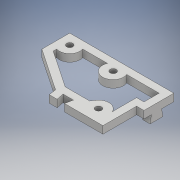
# Autodesk Inventor part: Frame VG01-1
Saved by Autodesk Inventor 2017 (Build 210142000, 142)
## iProperties
Created: 2019-03-04
Part Number: Frame VG01-1
Material: Generic
Document SubType Name: Modeling
Designer: Ben
Density: 1 g/cm^3
Appearance: Default
Author: Ben
Autodesk Inventor part; units mm, degrees
ref_plane "YZ Plane" through (0, 0, 0) normal (1, 0, 0) x (0, 1, 0)
ref_plane "XZ Plane" through (0, 0, 0) normal (0, 1, 0) x (-1, 0, 0)
ref_plane "XY Plane" through (0, 0, 0) normal (0, 0, 1) x (1, 0, 0)
sketch "Sketch1" plane through (0, 0, 0) normal (0, 1, 0) x (-1, 0, 0)
  line L0 (0, 0) -> (0, -35)
  line L1 (0, -35) -> (37, -35)
  line L2 (37, -35) -> (37, -55)
  line L3 (37, -55) -> (48, -55)
  line L4 (48, -55) -> (48, 0)
  line L5 (48, 0) -> (22, 0)
  line L6 (22, 0) -> (22, 0)
  line L7 (22, 0) -> (0, 0)
  dimension "d0" = 35
  dimension "d1" = 37
  dimension "d2" = 20
  dimension "d3" = 11
  dimension "d4" = 55
  dimension "d5" = 26
  dimension "d6" = 0
  constraints: 16 end point, 5 perpendicular, 2 vertical
  measures "d0" distance of L0.start L0.end
  measures "d1" distance of L0.end L1.end
  measures "d2" distance of L1.end L2.end
  measures "d3" distance of L2.end L3.end
  measures "d4" distance of L3.end L4.end
  measures "d5" distance of L4.end L5.end
  measures "d6" distance of L5.end L6.end
extrude "Extrusion1" add sketch "Sketch1" along normal blind 50
shell "Shell1" thickness 5 removed faces 3 at (-19.6667, 0, -23.3333) at (-48, 16.6667, -36.6667) at (-19.6667, 50, -23.3333)
sketch "Sketch2" plane through (0, 0, 0) normal (1, 0, 0) x (0, 0, -1)
  line L0 (5, 0) -> (30, 0) projected
  line L1 (5, 0) -> (19, 0)
  line L2 (19, 0) -> (19, 17)
  line L3 (19, 17) -> (5, 17)
  line L4 (5, 17) -> (5, 0)
  point P0 (0, 0)
  dimension "d10" = 17
  dimension "d11" = 0
  dimension "d12" = 11
  constraints: 8 end point, 2 parallel, 1 horizontal, 1 perpendicular, 1 point on line
  measures "d10" distance of L2.end L1.end
  measures "d11" distance from line of L4 L0.start
  measures "d12" distance from line of L2 L0.end
extrude "Extrusion2" cut sketch "Sketch2" against normal blind 10
sketch "Sketch3" plane through (-48, 0, -55) normal (-1, 0, 0) x (0, 0, 1)
  line L0 (0, 0) -> (0, 50) projected
  line L1 (5, 50) -> (25, 50) projected
  line L2 (0, 0) -> (5, 0)
  line L3 (5, 0) -> (5, 50)
  line L4 (5, 50) -> (0, 50)
  line L5 (0, 50) -> (0, 0)
  point P0 (55, 0)
  constraints: 8 end point, 2 parallel, 1 horizontal, 1 perpendicular
extrude "Extrusion3" add sketch "Sketch3" along normal blind 15
sketch "Sketch4" plane through (-48, 0, 0) normal (-1, 0, 0) x (0, 0, 1)
  line L0 (-5, 0) -> (0, 0) projected
  line L1 (-5, 0) -> (-5, 50) projected
  line L2 (0, 0) -> (-5, 0)
  line L3 (-5, 0) -> (-5, 50)
  line L4 (-5, 50) -> (0, 50)
  line L5 (0, 50) -> (0, 0)
  point P0 (0, 0)
  constraints: 8 end point, 2 parallel, 1 horizontal, 1 perpendicular
extrude "Extrusion4" add sketch "Sketch4" along normal blind 15
sketch "Sketch5" plane through (0, 17, -5) normal (0, 0, -1) x (-1, 0, 0)
  circle A0 centre (11.5, -8.5) radius 2.0828
  line L0 (63, -17) -> (0, -17) projected
  line L1 (0, -17) -> (0, 0) projected
  dimension "d19" = 4.1656
  dimension "d20" = 8.5
  dimension "d21" = 11.5
  constraints: 1 centre point
  measures "d19" diameter of A0
  measures "d20" distance from line of L0 A0.centre
  measures "d21" distance from line of L1 A0.centre
extrude "Extrusion5" cut sketch "Sketch5" against normal blind 15
sketch "Sketch6" plane through (0, 17, -5) normal (0, 0, -1) x (-1, 0, 0)
  circle A0 centre (28.505, 18.46) radius 2.0828
  line L0 (63, -17) -> (0, -17) projected
  line L1 (5, 0) -> (5, 33) projected
  dimension "d24" = 4.1656
  dimension "d25" = 35.46
  dimension "d26" = 23.505
  constraints: 1 centre point
  measures "d24" diameter of A0
  measures "d25" distance from line of L0 A0.centre
  measures "d26" distance from line of L1 A0.centre
extrude "Extrusion6" cut sketch "Sketch6" against normal blind 15
sketch "Sketch7" plane through (0, 17, -5) normal (0, 0, -1) x (-1, 0, 0)
  circle A0 centre (58.5, 19) radius 2.0828
  line L0 (63, 33) -> (63, -17) projected
  line L1 (5, 33) -> (63, 33) projected
  point P0 (0, -17)
  dimension "d29" = 4.1656
  dimension "d30" = 4.5
  dimension "d31" = 14
  constraints: 1 centre point
  measures "d29" diameter of A0
  measures "d30" distance from line of A0.centre L0
  measures "d31" distance from line of L1 A0.centre
extrude "Extrusion7" cut sketch "Sketch7" against normal blind 15
sketch "Sketch13" plane through (0, 0, -35) normal (0, 0, -1) x (-1, 0, 0)
  circle A0 centre (11.5, 8.5) radius 2.0828
  line L0 (0, 0) -> (37, 0) projected
  line L1 (0, 0) -> (0, 50) projected
  dimension "d41" = 4.1656
  dimension "d42" = 8.5
  dimension "d43" = 11.5
  constraints: 1 centre point
  measures "d41" diameter of A0
  measures "d42" distance from line of L0 A0.centre
  measures "d43" distance from line of L1 A0.centre
extrude "Extrusion9" cut sketch "Sketch13" against normal blind 15
sketch "Sketch14" plane through (-37, 0, -55) normal (0, 0, -1) x (-1, 0, 0)
  circle A0 centre (-8.495, 35.46) radius 2.0828
  line L0 (-37, 0) -> (-37, 50) projected
  line L1 (0, 0) -> (26, 0) projected
  dimension "d46" = 4.1656
  dimension "d47" = 28.505
  dimension "d48" = 35.46
  constraints: 1 centre point
  measures "d46" diameter of A0
  measures "d47" distance from line of L0 A0.centre
  measures "d48" distance from line of L1 A0.centre
extrude "Extrusion10" cut sketch "Sketch14" against normal blind 15
sketch "Sketch15" plane through (-37, 0, -55) normal (0, 0, -1) x (-1, 0, 0)
  circle A0 centre (21.5, 36) radius 2.0828
  line L0 (0, 0) -> (26, 0) projected
  line L1 (26, 50) -> (26, 0) projected
  point P0 (-37, 0)
  dimension "d51" = 4.1656
  dimension "d52" = 36
  dimension "d53" = 4.5
  constraints: 1 centre point
  measures "d51" diameter of A0
  measures "d52" distance from line of L0 A0.centre
  measures "d53" distance from line of L1 A0.centre
extrude "Extrusion11" cut sketch "Sketch15" against normal blind 15
sketch "Sketch16" plane through (-42, 0, -30) normal (-1, 0, 0) x (0, 0, 1)
  line L0 (0, 0) -> (-5, 0)
  line L1 (-5, 0) -> (-5, 50)
  line L2 (-5, 50) -> (0, 50)
  line L3 (0, 50) -> (0, 0)
  point P0 (30, 0)
  dimension "d56" = 5
  dimension "d57" = 50
  constraints: 8 end point, 2 parallel, 1 horizontal, 1 perpendicular
  measures "d56" distance of L1.end L2.end
  measures "d57" distance of L0.end L1.end
extrude "Extrusion12" add sketch "Sketch16" along normal blind 21
sketch "Sketch17" plane through (-5, 0, -30) normal (0, 0, 1) x (1, 0, 0)
  circle A0 centre (-23.505, 35.46) radius 2.0828
  line L0 (0, 0) -> (0, 50) projected
  line L1 (0, 0) -> (-58, 0) projected
  point P0 (5, 0)
  dimension "d60" = 4.1656
  dimension "d61" = 23.505
  dimension "d62" = 35.46
  constraints: 1 centre point
  measures "d60" diameter of A0
  measures "d61" distance from line of A0.centre L0
  measures "d62" distance from line of L1 A0.centre
extrude "Extrusion13" cut sketch "Sketch17" against normal blind 10
sketch "Sketch18" plane through (-42, 0, -35) normal (0, 0, -1) x (-1, 0, 0)
  circle A0 centre (16.5, 36) radius 2.0828
  line L0 (21, 50) -> (21, 0) projected
  line L1 (0, 0) -> (21, 0) projected
  point P0 (-42, 0)
  dimension "d65" = 4.1656
  dimension "d67" = 36
  dimension "d70" = 4.5
  constraints: 1 centre point
  measures "d65" diameter of A0
  measures "d67" distance from line of L1 A0.centre
  measures "d70" distance from line of L0 A0.centre
extrude "Extrusion14" cut sketch "Sketch18" against normal blind 10
sketch "Sketch20" plane through (-63, 0, 0) normal (-1, 0, 0) x (0, 0, 1)
  line L0 (0, 0) -> (-5, 0) projected
  line L1 (-5, 17) -> (-5, 50) projected
  line L2 (0, 0) -> (-5, 0)
  line L3 (-5, 0) -> (-5, 50)
  line L4 (-5, 50) -> (0, 50)
  line L5 (0, 50) -> (0, 0)
  constraints: 8 end point, 2 parallel, 1 horizontal, 1 perpendicular
extrude "Extrusion15" add sketch "Sketch20" along normal blind 2.583
sketch "Sketch21" plane through (-63, 0, -30) normal (-1, 0, 0) x (0, 0, 1)
  line L0 (-20, 50) -> (-5, 50) projected
  line L1 (11, 0) -> (0, 0) projected
  line L2 (-5, 50) -> (0, 50)
  line L3 (0, 50) -> (0, 0)
  line L4 (0, 0) -> (-5, 0)
  line L5 (-5, 0) -> (-5, 50)
  point P0 (30, 0)
  constraints: 8 end point, 2 parallel, 1 horizontal, 1 perpendicular
extrude "Extrusion16" add sketch "Sketch21" along normal blind 2.583
sketch "Sketch22" plane through (-63, 0, -55) normal (-1, 0, 0) x (0, 0, 1)
  line L0 (0, 0) -> (0, 50) projected
  line L1 (5, 0) -> (5, 50) projected
  line L2 (0, 50) -> (5, 50)
  line L3 (5, 50) -> (5, 0)
  line L4 (5, 0) -> (0, 0)
  line L5 (0, 0) -> (0, 50)
  point P0 (55, 0)
  constraints: 8 end point, 2 parallel, 1 horizontal, 1 perpendicular
extrude "Extrusion17" add sketch "Sketch22" along normal blind 2.583
sketch "Sketch23" plane through (0, 0, 0) normal (0, 0, 1) x (1, 0, 0)
  line L0 (0, 50) -> (-37, 50) projected
  line L1 (-65.583, 50) -> (-65.583, 0) projected
  line L2 (0, 50) -> (-65.583, 50)
  line L3 (-65.583, 50) -> (-65.583, 43.083)
  line L4 (-65.583, 43.083) -> (0, 43.083)
  line L5 (0, 43.083) -> (0, 50)
  point P0 (0, 0)
  dimension "d77" = 6.917
  constraints: 8 end point, 2 parallel, 1 horizontal, 1 perpendicular, 1 point on line
  measures "d77" distance of L4.end L0.start
extrude "Extrusion18" cut sketch "Sketch23" against normal blind 100
sketch "Sketch24" plane through (0, 0, -35) normal (0, 0, -1) x (-1, 0, 0)
  line L0 (0, 0) -> (65.583, 0) projected
  line L1 (31.0052, 0) -> (26.0052, 0)
  line L2 (26.0052, 5) -> (31.0052, 5)
  circle A0 centre (28.505, 35.46) radius 2.0828 projected
  line L3 (26.0052, 5) -> (25.0052, 5)
  line L4 (25.0052, 5) -> (26.0052, 0)
  line L5 (31.0052, 5) -> (32.0052, 5)
  line L6 (32.0052, 5) -> (31.0052, 0)
  dimension "d80" = 5
  dimension "d81" = 5
  dimension "d83" = 1
  dimension "d84" = 1
  constraints: 12 end point, 3 horizontal, 1 parallel, 1 point on line
  measures "d80" distance of L2.start L2.end
  measures "d81" distance of L1.end L2.start
  measures "d83" distance of L2.start L3.end
  measures "d84" distance of L2.end L5.end
extrude "Extrusion19" cut sketch "Sketch24" against normal blind 100 contours L4 L3 L2 L5 L6 L0
sketch "Sketch25" plane through (0, 0, 0) normal (1, 0, 0) x (0, 0, -1)
  line L0 (5, 0) -> (61.8537, 0)
  line L1 (61.8537, 0) -> (61.8537, 49.713)
  line L2 (61.8537, 49.713) -> (5, 49.713)
  line L3 (5, 49.713) -> (5, 0)
  line L4 (0, 0) -> (0, 43.083) projected
  dimension "d89" = 5
  constraints: 8 end point, 2 parallel, 1 horizontal, 1 perpendicular
  measures "d89" distance between parallel lines of L4 L3
extrude "Extrusion20" cut sketch "Sketch25" against normal blind 100
sketch "Sketch28" plane through (0, 0, 0) normal (1, 0, 0) x (0, 0, -1)
  line L0 (10, 43.083) -> (10, 17) projected
  line L1 (10, 35.6451) -> (10, 26.9508)
  line L2 (10, 26.9508) -> (5, 27.8324)
  line L3 (5, 43.083) -> (5, 0) projected
  line L4 (10, 35.6451) -> (5, 34.7635)
  line L5 (10, 35.6451) -> (15.0771, 35.6451) construction
  line L6 (5, 34.7635) -> (5, 27.8324)
  line L7 (10, 43.083) -> (10, 17) projected
  line L8 (5, 43.083) -> (0, 43.083) projected
  point P0 (0, 0)
  dimension "d111" = 8.6943
  dimension "d112" = 80
  dimension "d113" = 170
  dimension "d116" = 7.4379
  constraints: 10 end point, 3 point on line, 1 equal length, 1 horizontal, 1 parallel
  measures "d111" distance of L1.start L1.end
  measures "d112" angle of L1 L2
  measures "d113" angle of L4 L5
  measures "d116" distance from line of L8 L1.start
extrude "Extrusion22" add sketch "Sketch28" against normal blind 5
shell "Shell2" thickness 5 removed faces 2 at (-51.7832, 13.0175, 0) at (-51.7832, 13.0175, -5)
sketch "Sketch29" plane through (0, 43.083, -5) normal (0, 0, -1) x (-1, 0, 0)
  line L0 (38.1042, -33.083) -> (18.9062, -33.083) projected
  line L1 (18.9062, -33.083) -> (17.5166, -30.8459)
  arc A0 (17.6576, -38.083) -> (5, -31.7695) centre (11.5, -34.583) ccw projected
  line L2 (18.9062, -33.083) -> (22.5612, -39.2148)
  line L3 (22.5612, -39.2148) -> (2.6818, -40.5517)
  line L4 (2.6818, -40.5517) -> (3.5455, -34.2971)
  line L5 (3.5455, -34.2971) -> (13.8172, -38.9728)
  line L6 (13.8172, -38.9728) -> (17.5166, -30.8459)
  point P0 (0, -43.083)
  constraints: 12 end point, 1 perpendicular, 1 point on circle, 1 tangent
extrude "Extrusion23" add sketch "Sketch29" against normal blind 5
sketch "Sketch30" plane through (0, 0, 0) normal (1, 0, 0) x (0, 0, -1)
  line L0 (5, 43.083) -> (0, 43.083) projected
  line L1 (0, 43.083) -> (0, 22.8324)
  line L2 (0, 0) -> (0, 43.083) projected
  line L3 (0, 22.8324) -> (5, 22.8324)
  line L4 (5, 11.3135) -> (5, 27.8324) projected
  line L5 (5, 27.8324) -> (5, 22.8324)
  line L6 (10, 26.9508) -> (5, 27.8324) projected
  line L7 (5, 27.8324) -> (10, 26.9508)
  line L8 (10, 26.9508) -> (10, 35.6451) projected
  line L9 (10, 26.9508) -> (10, 35.6451)
  line L10 (10, 35.6451) -> (5, 34.7635) projected
  line L11 (10, 35.6451) -> (5, 34.7635)
  line L12 (5, 34.7635) -> (5, 43.083)
  line L13 (0, 43.083) -> (5, 43.083)
  dimension "d123" = 5
  constraints: 16 end point, 3 collinear, 2 perpendicular, 2 point on line, 1 horizontal, 1 parallel
  measures "d123" distance from line of L3 L4.end
extrude "Extrusion24" add sketch "Sketch30" along normal blind 5
sketch "Sketch31" plane through (-65.583, 0, 0) normal (0, 0, 1) x (1, 0, 0)
  line L0 (60.583, 38.083) -> (65.583, 38.083)
  line L1 (65.583, 38.083) -> (65.583, 27.8324)
  line L2 (65.583, 27.8324) -> (60.583, 27.8324)
  line L3 (60.583, 27.8324) -> (60.583, 38.083)
  line L4 (70.583, 43.083) -> (70.583, 22.8324) projected
  line L5 (65.583, 22.8324) -> (70.583, 22.8324) projected
  line L6 (70.583, 43.083) -> (0, 43.083) projected
  point P0 (65.583, 0)
  dimension "d124" = 5
  dimension "d125" = 5
  dimension "d126" = 5
  dimension "d127" = 5
  constraints: 8 end point, 2 parallel, 1 horizontal, 1 perpendicular
  measures "d124" distance between parallel lines of L4 L1
  measures "d125" distance between parallel lines of L5 L2
  measures "d126" distance of L0.start L0.end
  measures "d127" distance between parallel lines of L6 L0
extrude "Extrusion25" cut sketch "Sketch31" against normal blind 15
sketch "Sketch32" plane through (-5, 27.8324, -5) normal (0, 1, 0) x (1, 0, 0)
  line L0 (0, 5) -> (0, 0) projected
  line L1 (0, 0) -> (5, 0)
  line L2 (5, 0) -> (5, 5)
  line L3 (5, 5) -> (0, 5)
  line L4 (0, 5) -> (0, 0)
  point P0 (5, -5)
  dimension "d130" = 5
  dimension "d131" = 5
  constraints: 8 end point, 2 parallel, 1 horizontal, 1 perpendicular
  measures "d130" distance of L3.end L2.end
  measures "d131" distance of L2.end L1.end
extrude "Extrusion26" cut sketch "Sketch32" against normal blind 15
sketch "Sketch33" plane through (-65.583, 0, 0) normal (0, 0, 1) x (1, 0, 0)
  line L0 (5, 29.2304) -> (5, 5) projected
  line L1 (5, 29.2304) -> (0, 24.2304)
  line L2 (0, 0) -> (0, 43.083) projected
  line L3 (5, 29.2304) -> (12.0711, 29.2304) construction
  line L4 (34.5778, 0) -> (0, 0) projected
  line L5 (0, 24.2304) -> (0, 0)
  line L6 (0, 0) -> (29.2304, 0)
  line L7 (28.4788, 5) -> (5, 29.2304)
  line L8 (28.4788, 5) -> (29.2304, 0)
  point P0 (65.583, 0)
  dimension "d134" = 135
  constraints: 12 end point, 2 point on line, 1 equal length, 1 horizontal, 1 perpendicular
  measures "d134" angle of L1 L3
extrude "Extrusion27" cut sketch "Sketch33" against normal blind 10
sketch "Sketch34" plane through (-26.0052, 0, 0) normal (0, 0, 1) x (1, 0, 0)
  line L0 (-10.3474, 0) -> (-11.099, 5) projected
  line L1 (-10.3474, 0) -> (-12.1235, 11.8152)
  line L2 (-12.1235, 11.8152) -> (-14.1606, 7.7448)
  line L3 (-14.1606, 7.7448) -> (-10.3474, 0)
  point P0 (26.0052, 0)
  constraints: 6 end point, 1 collinear
extrude "Extrusion28" cut sketch "Sketch34" against normal blind 10
sketch "Sketch35" plane through (-26.0052, 0, 0) normal (0, 0, 1) x (1, 0, 0)
  line L0 (-39.5778, 24.2304) -> (-34.5778, 29.2304) projected
  line L1 (-39.5778, 24.2304) -> (-11.099, 5)
  line L2 (-11.8507, 10) -> (-10.3474, 0) projected
  line L3 (-11.099, 5) -> (-8.3009, 9.1438)
  line L4 (-8.3009, 9.1438) -> (-35.9765, 27.8318)
  point P0 (26.0052, 0)
  dimension "d139" = 5
  constraints: 6 end point, 1 midpoint, 1 parallel, 1 perpendicular, 1 point on line
  measures "d139" distance of L1.end L3.end
extrude "Extrusion29" add sketch "Sketch35" against normal blind 5
sketch "Sketch36" plane through (-26.0052, 0, 0) normal (0, 0, 1) x (1, 0, 0)
  line L0 (-39.5486, 28.0765) -> (-34.5486, 28.0765) construction
  line L1 (-34.5486, 28.0765) -> (-34.5486, 26.0112)
  line L2 (-34.5486, 26.0112) -> (-37.3456, 26.0112)
  line L3 (-37.3456, 26.0112) -> (-37.3456, 30.6925)
  line L4 (-37.3456, 30.6925) -> (-34.5486, 30.6925)
  line L5 (-34.5486, 30.6925) -> (-34.5486, 28.0765)
  point P0 (26.0052, 0)
  dimension "d142" = 5
  constraints: 12 end point, 4 perpendicular, 1 horizontal, 1 point on line, 1 vertical
  measures "d142" distance of L0.start L0.end
extrude "Extrusion30" add sketch "Sketch36" against normal blind 5
body "Solid1"
